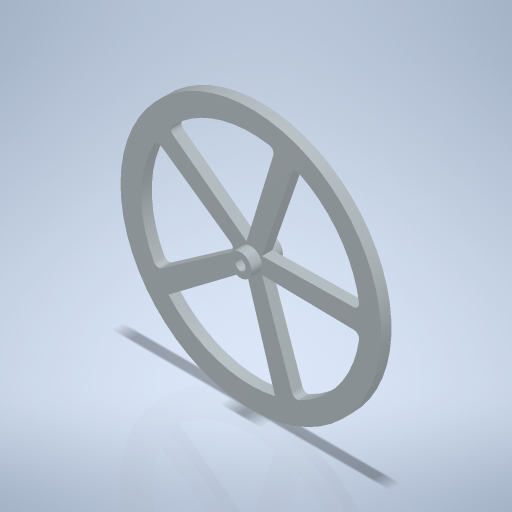
# Autodesk Inventor part: wheel
Saved by Autodesk Inventor 2024 (Build 280153000, 153)
## iProperties
Created: 2024-06-06
Part Number: wheel
Material: Aluminium 6061
Document SubType Name: Modeling
Designer: ffogue
Density: 2.7 g/cm^3
Appearance: Zink
Author: ffogue
Autodesk Inventor part; units mm, degrees
note: some values were not read from the file. Chosen so that the rebuilt part matches the saved one: direction of "Bohrung1".
ref_plane "YZ Plane" through (0, 0, 0) normal (1, 0, 0) x (0, 1, 0)
ref_plane "XY Plane" through (0, 0, 0) normal (0, 0, 1) x (1, 0, 0)
sketch "Skizze1" plane through (0, 0, 0) normal (0, 1, 0) x (-1, 0, 0)
  circle A0 centre (0, 0) radius 75
  dimension "d0" = 150
  constraints: 1 centre point, 1 coincident
  measures "d0" diameter of A0
extrude "Extrusion1" add sketch "Skizze1" along normal mid plane 6
ref_plane "Arbeitsebene1" through (0, 0, 0) normal (0, 1, 0) x (-1, 0, 0)
sketch "Skizze4" plane through (0, 0, 0) normal (0, 1, 0) x (-1, 0, 0)
  circle A0 centre (0, 0) radius 6.5
  dimension "d17" = 13
  constraints: 1 centre point, 1 coincident
  measures "d17" diameter of A0
extrude "Extrusion3" add sketch "Skizze4" along normal mid plane 18
sketch "Skizze5" plane through (0, 9, 0) normal (0, 1, 0) x (1, 0, 0)
  circle A0 centre (0, 0) radius 6.5 projected
  constraints: 1 coincident
hole "Bohrung1" at (0, 9, 0) direction (0, -1, 0) diameter 6 end up to surface
sketch "Skizze2" plane through (0, 3, 0) normal (0, 1, 0) x (1, 0, 0)
  circle A0 centre (0, 0) radius 63 construction
  circle A1 centre (0, 0) radius 75 projected
  line L0 (0, 0) -> (0, -75) construction
  line L1 (0, 0) -> (-75, 0) construction
  circle A2 centre (0, 0) radius 6.5 projected
  line L2 (-8, 0) -> (-54.1014, -32.2806)
  line L3 (-8, 0) -> (-54.1014, 32.2806)
  arc A3 (-54.1014, 32.2806) -> (-54.1014, -32.2806) centre (0, 0) ccw
  dimension "d3" = 126
  dimension "d40" = 8
  dimension "d41" = 35
  constraints: 8 end point, 6 point on circle, 2 centre point, 1 coincident, 1 concentric, 1 perpendicular, 1 point on line, 1 symmetric about line, 1 vertical
  measures "d3" diameter of A0
  measures "d40" distance of point (0, 0) L2.start
  measures "d41" angle of L1 L2
extrude "Extrusion2" cut sketch "Skizze2" against normal up to surface (6 mm away) contours L2 A3 L3
fillet "Rundung1" radius 3 3 edges at (-8, 0, 0) (-54.1014, 0, 32.2806) (-54.1014, 0, -32.2806)
pattern_circular "Runde Anordnung3" count 5 over 360 about axis through (0, 0, 0) along (0, 1, 0) of "Extrusion2"
fillet "Rundung3" radius 3 6 edges at (24.7949, 0, -57.9156) (62.743, 0, -5.6845) (62.743, 0, 5.6845) (24.7949, 0, 57.9156) (13.9824, 0, 61.4288) (-47.4189, 0, 41.4783)
